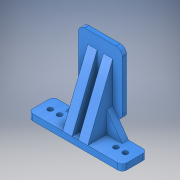
# Autodesk Inventor part: Mordaza
Saved by Autodesk Inventor 2019 (Build 230136000, 136)
## iProperties
Created: 2020-04-03
Part Number: Mordaza
Material: Generic
Document SubType Name: Modeling
Designer: Jurgen
Density: 1 g/cm^3
Appearance: Cyan
Mass: 174.718 g
Surface Area: 416.169 cm^2
Volume: 174.718 cm^3
Author: Jurgen
Autodesk Inventor part; units mm, degrees
ref_plane "YZ Plane" through (0, 0, 0) normal (1, 0, 0) x (0, 1, 0)
ref_plane "XZ Plane" through (0, 0, 0) normal (0, 1, 0) x (-1, 0, 0)
sketch "Sketch1" plane through (0, 0, 0) normal (0, 0, 1) x (1, 0, 0)
  line L0 (35, -50) -> (-35, -50)
  line L1 (-35, -50) -> (-35, 50)
  line L2 (-35, 50) -> (35, 50)
  line L3 (35, 50) -> (35, -50)
  line L4 (35, -50) -> (-35, 50) construction
  line L5 (-35, -50) -> (35, 50) construction
  point P0 (0, 0)
  dimension "d0" = 70
  dimension "d1" = 100
  constraints: 12 end point, 2 midpoint, 2 parallel, 1 horizontal, 1 perpendicular
  measures "d0" distance of L1.end L2.end
  measures "d1" distance of L0.end L1.end
extrude "Extrusion1" add sketch "Sketch1" along normal blind 7
fillet "Fillet1" radius 10 4 edges at (35, 50, 3.5) (-35, 50, 3.5) (-35, -50, 3.5) (35, -50, 3.5)
ref_plane "Work Plane1" through (-20, -40, 0) normal (-1, 0, 0) x (0, 0, 1)
sketch "Sketch2" plane through (-20, -40, 0) normal (-1, 0, 0) x (0, 0, 1)
  line L0 (7, 80) -> (7, 90) construction
  line L1 (7, 90) -> (0, 90) construction
  line L2 (0, 90) -> (0, 80) construction
  line L3 (0, 80) -> (7, 80) construction
  line L4 (7, 0) -> (0, 0) construction
  line L5 (7, 80) -> (7, 0) construction
  line L6 (0, 80) -> (7, 80) construction
  line L7 (0, 0) -> (0, 80) construction
  line L8 (7, -10) -> (7, 0) construction
  line L9 (7, 0) -> (0, 0) construction
  line L10 (0, 0) -> (0, -10) construction
  line L11 (0, -10) -> (7, -10) construction
  line L12 (0, -10) -> (7, -10) construction
  line L13 (57, 70) -> (7, 70) construction
  line L14 (7, 70) -> (7, -10) construction
  line L15 (7, 70) -> (47, 70) construction
  line L16 (47, 70) -> (47, -30) construction
  line L17 (47, -30) -> (7, -30) construction
  line L18 (7, -30) -> (7, 70) construction
  line L19 (7, 70) -> (7, -30)
  line L20 (7, -30) -> (47, -30)
  line L21 (47, -30) -> (7, 70)
  line L22 (0, 0) -> (7, 0) construction
  line L23 (0, 80) -> (0, 0) construction
  line L24 (7, 80) -> (0, 80) construction
  line L25 (7, 0) -> (7, 80) construction
  line L26 (7, 90) -> (7, 80) construction
  line L27 (7, 80) -> (0, 80) construction
  line L28 (0, 80) -> (0, 90) construction
  line L29 (0, 90) -> (7, 90) construction
  line L30 (7, 0) -> (7, -10) construction
  line L31 (7, -10) -> (0, -10) construction
  line L32 (0, -10) -> (0, 0) construction
  line L33 (0, 0) -> (7, 0) construction
  point P0 (0, 40)
  dimension "d6" = 50
  dimension "d8" = 40
  dimension "d9" = 100
  dimension "d17" = 20
  constraints: 18 end point, 3 equal length, 2 perpendicular, 1 horizontal
  measures "d6" distance of L13.end L13.start
  measures "d8" distance of L16.end L17.end
  measures "d9" distance of L15.end L16.end
  measures "d17" distance between parallel lines of L1 L15
extrude "Extrusion2" add sketch "Sketch2" against normal blind 40
sketch "Sketch3" plane through (-20, -70, 7) normal (0, -1, 0) x (1, 0, 0)
  line L0 (0, 0) -> (0, 40) construction
  line L1 (0, 0) -> (40, 0) construction
  line L2 (40, 40) -> (40, 0) construction
  line L3 (0, 40) -> (40, 40) construction
  line L4 (0, 40) -> (-55, 40) construction
  line L5 (-55, 40) -> (95, 40)
  line L6 (95, 40) -> (95, 0)
  line L7 (95, 0) -> (-55, 0)
  line L8 (-55, 0) -> (-55, 40)
  point P0 (20, -7)
  dimension "d12" = 55
  dimension "d13" = 150
  dimension "d18" = 40
  constraints: 10 end point, 2 parallel, 1 horizontal, 1 perpendicular, 1 point on line
  measures "d12" distance of L0.end L4.end
  measures "d13" distance of L6.end L7.end
  measures "d18" distance of L7.end L4.end
extrude "Extrusion3" add sketch "Sketch3" along normal blind 10
fillet "Fillet2" radius 7 4 edges at (-75, -75, 47) (75, -75, 47) (75, -75, 7) (-75, -75, 7)
sketch "Sketch5" plane through (-20, -80, 7) normal (0, -1, 0) x (1, 0, 0)
  arc A0 (-55, 7) -> (-48, 0) centre (-48, 7) ccw construction
  line L0 (-48, 0) -> (88, 0) construction
  arc A1 (88, 0) -> (95, 7) centre (88, 7) ccw construction
  line L1 (95, 7) -> (95, 33) construction
  arc A2 (95, 33) -> (88, 40) centre (88, 33) ccw construction
  line L2 (88, 40) -> (-48, 40) construction
  arc A3 (-48, 40) -> (-55, 33) centre (-48, 33) ccw construction
  line L3 (-55, 33) -> (-55, 7) construction
  line L4 (95, 20) -> (-55, 20) construction
  line L5 (-55, 7) -> (-55, 33) construction
  line L6 (0, 0) -> (40, 0) construction
  line L7 (20, 0) -> (20, 40) construction
  circle A4 centre (80, 20) radius 4
  circle A5 centre (-40, 20) radius 4
  circle A6 centre (65, 20) radius 4
  circle A7 centre (-25, 20) radius 4
  point P0 (20, -7)
  dimension "d23" = 8
  dimension "d24" = 8
  dimension "d25" = 15
  dimension "d26" = 15
  dimension "d29" = 8
  dimension "d30" = 8
  dimension "d31" = 15
  dimension "d32" = 15
  constraints: 4 centre point, 4 end point, 4 midpoint, 4 point on line
  measures "d23" diameter of A4
  measures "d24" diameter of A5
  measures "d25" distance from line of L1 A4.centre
  measures "d26" distance of L4.end A5.centre
  measures "d29" diameter of A6
  measures "d30" diameter of A7
  measures "d31" distance of A4.centre A6.centre
  measures "d32" distance of A7.centre A5.centre
extrude "Extrusion4" cut sketch "Sketch5" against normal blind 20
sketch "Sketch7" plane through (-20, -70, 47) normal (0, 0, 1) x (1, 0, 0)
  line L0 (0, 0) -> (0, 100) construction
  line L1 (0, 0) -> (40, 0) construction
  line L2 (40, 100) -> (40, 0) construction
  line L3 (0, 100) -> (40, 100) construction
  line L4 (20, 100) -> (20, 0) construction
  line L5 (0, 20) -> (0, 100) construction
  line L6 (0, 50) -> (20, 50) construction
  line L7 (25, 0) -> (15, 0)
  line L8 (15, 0) -> (15, 100)
  line L9 (15, 100) -> (25, 100)
  line L10 (25, 100) -> (25, 0)
  line L11 (25, 0) -> (15, 100) construction
  line L12 (15, 0) -> (25, 100) construction
  point P0 (20, 70)
  dimension "d33" = 10
  constraints: 16 end point, 5 midpoint, 2 parallel, 2 point on line, 1 horizontal, 1 perpendicular
  measures "d33" distance of L8.end L9.end
extrude "Extrusion5" cut sketch "Sketch7" against normal blind 40
sketch "Sketch8" plane through (0, 0, 7) normal (0, 0, 1) x (1, 0, 0)
  line L0 (-20, -50) -> (-20, 30) construction
  line L1 (-20, 30) -> (-5, 30) construction
  line L2 (-5, -50) -> (-5, 30) construction
  line L3 (-5, -50) -> (5, -50) construction
  line L4 (5, 30) -> (5, -50) construction
  line L5 (5, 30) -> (20, 30) construction
  line L6 (20, 30) -> (20, -50) construction
  line L7 (20, -50) -> (25, -50) construction
  arc A0 (25, -50) -> (35, -40) centre (25, -40) ccw construction
  line L8 (35, -40) -> (35, 40) construction
  arc A1 (35, 40) -> (25, 50) centre (25, 40) ccw construction
  line L9 (25, 50) -> (-25, 50) construction
  arc A2 (-25, 50) -> (-35, 40) centre (-25, 40) ccw construction
  line L10 (-35, 40) -> (-35, -40) construction
  arc A3 (-35, -40) -> (-25, -50) centre (-25, -40) ccw construction
  line L11 (-25, -50) -> (-20, -50) construction
  line L12 (-5, -70) -> (-5, 30) construction
  line L13 (-20, 30) -> (-5, 30) construction
  line L14 (-20, -70) -> (-20, 30) construction
  line L15 (-20, -70) -> (-5, -70) construction
  line L16 (5, 30) -> (5, -70) construction
  line L17 (5, -70) -> (20, -70) construction
  line L18 (20, 30) -> (20, -70) construction
  line L19 (5, 30) -> (20, 30) construction
  line L20 (68, -70) -> (68, -80) construction
  line L21 (20, -70) -> (68, -70) construction
  line L22 (5, -70) -> (20, -70) construction
  line L23 (-5, -70) -> (5, -70) construction
  line L24 (-20, -70) -> (-5, -70) construction
  line L25 (-68, -70) -> (-20, -70) construction
  line L26 (-68, -80) -> (-68, -70) construction
  line L27 (68, -80) -> (-68, -80) construction
  line L28 (-20, -70) -> (-45, -70)
  line L29 (-20, -70) -> (-20, -35)
  line L30 (-20, -35) -> (-45, -70)
  line L31 (25, -50) -> (-25, -50) construction
  line L32 (0, -50) -> (0, -70) construction
  line L33 (20, -70) -> (45, -70)
  line L34 (20, -70) -> (20, -35)
  line L35 (20, -35) -> (45, -70)
  point P0 (0, 0)
  dimension "d0" = 70
  dimension "d36" = 25
  dimension "d37" = 35
  constraints: 14 end point, 3 symmetric about line, 2 midpoint, 2 point on line
  measures "d36" distance of L24.start L28.end
  measures "d37" distance of L24.start L29.end
extrude "Extrusion6" add sketch "Sketch8" along normal blind 10
body "Solid1"
